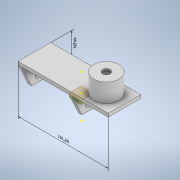
# Autodesk Inventor part: angleadjuster
Saved by Autodesk Inventor 2020.1 (Build 241239000, 239)
## iProperties
Created: 2019-11-07
Part Number: angleadjuster
Material: Generic
Document SubType Name: Modeling
Designer: super
Density: 1 g/cm^3
Appearance: Default
Author: super
Autodesk Inventor part; units mm, degrees
ref_plane "YZ Plane" through (0, 0, 0) normal (1, 0, 0) x (0, 1, 0)
ref_plane "XZ Plane" through (0, 0, 0) normal (0, 1, 0) x (-1, 0, 0)
ref_plane "XY Plane" through (0, 0, 0) normal (0, 0, 1) x (1, 0, 0)
ref_plane "Work Plane3" through (0, 6, 0) normal (0, 1, 0) x (1, 0, 0)
sketch "Sketch2" plane through (0, 6, 0) normal (0, 1, 0) x (1, 0, 0)
  line L0 (0, 0) -> (0, 22.5)
  line L1 (0, 45) -> (0, 0) projected
  line L2 (0, 22.5) -> (22.5, 22.5)
  circle A0 centre (22.5, 22.5) radius 22.5
  dimension "d5" = 22.5
  dimension "d6" = 22.5
  dimension "d7" = 45
  constraints: 4 end point, 1 centre point, 1 coincident, 1 midpoint, 1 perpendicular
  measures "d5" distance of L0.start L0.end
  measures "d6" distance of L0.end L2.end
  measures "d7" diameter of A0
extrude "Extrusion2" add sketch "Sketch2" along normal blind 33.5
ref_plane "Work Plane2" through (0, 0, 0) normal (0, -1, 0) x (1, 0, 0)
sketch "Sketch3" plane through (0, 0, 0) normal (0, -1, 0) x (1, 0, 0)
  line L0 (0, -45) -> (0, 0) projected
  line L1 (0, 0) -> (0, -22.5)
  circle A0 centre (22.5, -22.5) radius 18.25
  dimension "d12" = 36.5
  constraints: 2 end point, 1 centre point, 1 midpoint
  measures "d12" diameter of A0
extrude "Extrusion3" cut sketch "Sketch3" against normal blind 65
sketch "Sketch4" plane through (22.5, 39.5, -22.5) normal (0, 1, 0) x (1, 0, 0)
  circle A0 centre (0, 0) radius 6.75
  point P0 (-22.5, -22.5)
  dimension "d15" = 13.5
  constraints: 1 centre point
  measures "d15" diameter of A0
extrude "Extrusion4" cut sketch "Sketch4" against normal blind 4.5
ref_plane "Work Plane1" through (0, 0, 0) normal (0, -1, 0) x (1, 0, 0)
sketch "Sketch5" plane through (0, 0, 0) normal (0, -1, 0) x (1, 0, 0)
  line L0 (0, -45) -> (0, 0) projected
  line L1 (0, 0) -> (22.5, 0)
  line L2 (0, 0) -> (45, 0) projected
  constraints: 2 end point, 1 midpoint
sketch "Sketch6" plane through (22.5, 39.5, -22.5) normal (0, 1, 0) x (1, 0, 0)
  point P0 (-22.5, -22.5)
sketch "Sketch7" plane through (22.5, 39.5, -22.5) normal (0, 1, 0) x (1, 0, 0)
  circle A0 centre (0, 0) radius 18.25 projected
  circle A1 centre (0, 0) radius 18.25
  point P0 (-22.5, -22.5)
  constraints: 1 centre point, 1 coincident
extrude "Extrusion5" add sketch "Sketch7" against normal blind 3.5
sketch "Sketch8" plane through (22.5, 39.5, -22.5) normal (0, 1, 0) x (1, 0, 0)
  circle A0 centre (0, 0) radius 6.75
  point P0 (-22.5, -22.5)
  dimension "d20" = 13.5
  constraints: 1 centre point
  measures "d20" diameter of A0
extrude "Extrusion6" cut sketch "Sketch8" against normal blind 3.5
sketch "Sketch9" plane through (22.5, 6, -22.5) normal (0, -1, 0) x (1, 0, 0)
  point P0 (-22.5, 22.5)
sketch "Sketch10" plane through (22.5, 39.5, -22.5) normal (0, 1, 0) x (1, 0, 0)
  point P0 (-22.5, -22.5)
sketch "Sketch11" plane through (22.5, 6, -22.5) normal (0, -1, 0) x (1, 0, 0)
  circle A0 centre (0, 0) radius 22.5 projected
  line L0 (0, 29) -> (32.5, 29)
  line L1 (32.5, 29) -> (32.5, -29)
  line L2 (32.5, -29) -> (-32.5, -29)
  line L3 (0, 29) -> (-32.5, 29)
  line L4 (-32.5, -29) -> (-128.5, -29)
  line L5 (-128.5, -29) -> (-128.5, 29)
  line L6 (-128.5, 29) -> (-32.5, 29)
  point P0 (-22.5, 22.5)
  dimension "d25" = 58
  dimension "d26" = 65
  dimension "d27" = 32.5
  dimension "d28" = 96
  constraints: 14 end point, 5 perpendicular, 1 horizontal
  measures "d25" distance of L0.end L1.end
  measures "d26" distance of L1.end L2.end
  measures "d27" distance of L0.start L3.end
  measures "d28" distance of L2.end L4.end
sketch "Sketch12" plane through (22.5, 6, -22.5) normal (0, -1, 0) x (1, 0, 0)
  point P0 (-22.5, 22.5)
extrude "Extrusion7" add sketch "Sketch11" along normal blind 6
sketch "Sketch13" plane through (22.5, 6, -22.5) normal (0, -1, 0) x (1, 0, 0)
  circle A0 centre (0, 0) radius 6.75 projected
  circle A1 centre (0, 0) radius 22.5
  point P0 (-22.5, 22.5)
  constraints: 1 centre point, 1 coincident
extrude "Extrusion8" add sketch "Sketch13" along normal blind 6 contours A0 | A1
sketch "Sketch14" plane through (22.5, 0, -22.5) normal (0, -1, 0) x (1, 0, 0)
  circle A0 centre (0, 0) radius 18.25
  point P0 (-22.5, 22.5)
  constraints: 1 centre point
extrude "Extrusion9" cut sketch "Sketch14" against normal blind 6
sketch "Sketch15" plane through (-106, 6, -51.5) normal (-1, 0, 0) x (0, 0, 1)
  line L0 (58, -6) -> (0, -6) projected
  line L1 (29, -42) -> (38, -42)
  line L2 (29, -42) -> (20, -42)
  line L3 (20, -42) -> (0, -6)
  line L4 (38, -42) -> (58, -6)
  circle A0 centre (29, -33) radius 5
  point P0 (51.5, -6)
  dimension "d38" = 18
  dimension "d41" = 10
  constraints: 8 end point, 1 centre point, 1 horizontal
  measures "d38" distance of L1.end L2.end
  measures "d41" diameter of A0
extrude "Extrusion10" add sketch "Sketch15" against normal blind 6
sketch "Sketch17" plane through (-106, -36, -31.5) normal (0, -1, 0) x (1, 0, 0)
  point P0 (106, 31.5)
sketch "Sketch18" plane through (-106, -36, -31.5) normal (0, -1, 0) x (1, 0, 0)
  line L0 (6, 18) -> (6, 0) projected
  line L1 (6, 18) -> (0, 18)
  line L2 (0, 38) -> (0, -20) projected
  line L3 (0, 0) -> (6, 0)
  line L4 (6, 0) -> (6, 18)
  line L5 (0, 18) -> (0, 0)
  point P0 (106, 31.5)
  constraints: 8 end point, 2 horizontal, 1 parallel, 1 perpendicular, 1 point on line
extrude "Extrusion12" add sketch "Sketch18" along normal blind 2
sketch "Sketch19" plane through (-106, 6, -51.5) normal (-1, 0, 0) x (0, 0, 1)
  line L0 (38, -42) -> (38, -44) projected
  line L1 (38, -44) -> (40, -44)
  line L2 (58, -44) -> (0, -44) projected
  line L3 (38, -42) -> (58, -6) projected
  line L4 (40, -44) -> (58, -6)
  line L5 (58, -6) -> (38, -42)
  line L6 (38, -42) -> (38, -44)
  line L7 (40, -44) -> (38, -44)
  point P0 (51.5, -6)
  dimension "d53" = 2
  constraints: 10 end point, 2 perpendicular, 1 collinear, 1 point on line
  measures "d53" distance of L0.end L1.end
extrude "Extrusion13" add sketch "Sketch19" against normal blind 6
sketch "Sketch20" plane through (-106, 6, -51.5) normal (-1, 0, 0) x (0, 0, 1)
  line L0 (20, -42) -> (20, -44) projected
  line L1 (20, -44) -> (18, -44)
  line L2 (58, -44) -> (0, -44) projected
  line L3 (0, -6) -> (20, -42) projected
  line L4 (18, -44) -> (0, -6)
  line L5 (0, -6) -> (20, -42)
  line L6 (20, -42) -> (20, -44)
  line L7 (18, -44) -> (20, -44)
  point P0 (51.5, -6)
  dimension "d56" = 2
  constraints: 10 end point, 2 perpendicular, 1 collinear, 1 point on line
  measures "d56" distance of L0.end L1.end
extrude "Extrusion14" add sketch "Sketch20" against normal blind 6
sketch "Sketch24" plane through (55, 6, -51.5) normal (0, 0, -1) x (-1, 0, 0)
  line L0 (155, -6) -> (0, -6) projected
  point P0 (55, -6)
  point P1 (61, -6)
sketch "Sketch25" plane through (22.5, 0, -22.5) normal (0, -1, 0) x (1, 0, 0)
  line L0 (-32.5, -29) -> (-38.5, -29)
  line L1 (-38.5, -29) -> (-38.5, 29)
  line L2 (32.5, 29) -> (-122.5, 29) projected
  line L3 (-38.5, 29) -> (-32.5, 29)
  line L4 (-32.5, 29) -> (-32.5, -29)
  point P0 (-22.5, 22.5)
  dimension "d71" = 6
  dimension "d72" = 6
  constraints: 8 end point, 2 perpendicular, 1 point on line
  measures "d71" distance of L0.start L0.end
  measures "d72" distance of L1.end L3.end
extrude "Extrusion18" add sketch "Sketch25" along normal blind 38
sketch "Sketch26" plane through (-10, 0, 6.5) normal (1, 0, 0) x (0, 0, -1)
  line L0 (0, 0) -> (58, 0) projected
  circle A0 centre (29, -27) radius 5
  point P0 (6.5, 0)
  dimension "d76" = 10
  constraints: 1 centre point
  measures "d76" diameter of A0
sketch "Sketch27" plane through (-10, 0, 6.5) normal (1, 0, 0) x (0, 0, -1)
  point P0 (6.5, 0)
extrude "Extrusion19" cut sketch "Sketch26" against normal blind 6
sketch "Sketch28" plane through (-10, 0, 6.5) normal (1, 0, 0) x (0, 0, -1)
  circle A0 centre (29, -27) radius 5 projected
  line L0 (58, 0) -> (58, -38) projected
  line L1 (40, -38) -> (58, 0)
  line L2 (58, 0) -> (58, -38)
  line L3 (58, -38) -> (40, -38)
  point P0 (6.5, 0)
  constraints: 6 end point, 1 perpendicular
extrude "Extrusion20" cut sketch "Sketch28" against normal blind 6 contours L0 L3 L1
sketch "Sketch29" plane through (-10, -38, 6.5) normal (1, 0, 0) x (0, 0, -1)
  circle A0 centre (29, 11) radius 5 projected
  line L0 (0, 38) -> (18, 0) projected
  line L1 (18, 0) -> (0, 38)
  line L2 (0, 38) -> (0, 0) projected
  line L3 (0, 38) -> (0, 0)
  line L4 (0, 0) -> (18, 0)
  point P0 (6.5, 38)
  constraints: 6 end point, 2 collinear, 1 perpendicular
extrude "Extrusion21" cut sketch "Sketch29" against normal blind 6 contours L0 L4 L2
sketch "Sketch30" plane through (55, 6, -51.5) normal (0, 0, -1) x (-1, 0, 0)
  point P0 (55, -6)
body "Solid1"
